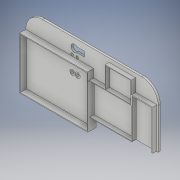
# Autodesk Inventor part: Base Plate 2
Saved by Autodesk Inventor 2018 (Build 220112000, 112)
## iProperties
Created: 2018-06-13
Part Number: Base Plate 2
Material: Generic
Document SubType Name: Modeling
Designer: brend
Density: 1 g/cm^3
Appearance: Default
Author: brend
Autodesk Inventor part; units mm, degrees
sketch "Sketch1" plane through (0, 0, 0) normal (0, 0, 1) x (1, 0, 0)
  line L0 (0, 87.3125) -> (163.83, 87.3125)
  line L1 (163.83, 87.3125) -> (163.83, 0)
  line L2 (163.83, 0) -> (0, 0)
  line L3 (0, 0) -> (0, 87.3125)
  dimension "d0" = 163.83
  dimension "d1" = 87.3125
  constraints: 8 end point, 2 parallel, 1 horizontal, 1 perpendicular
  measures "d0" distance between parallel lines of L1 L3
  measures "d1" distance between parallel lines of L2 L0
extrude "Extrusion1" add sketch "Sketch1" along normal blind 2.54
sketch "Sketch2" plane through (0, 0, 2.54) normal (0, 0, 1) x (1, 0, 0)
  point P0 (0, 0)
fillet "Fillet1" radius 20.6375 1 edges at (163.83, 87.3125, 1.27)
fillet "Fillet2" radius 20.6375 1 edges at (0, 87.3125, 1.27)
sketch "Sketch8" plane through (0, 0, 2.54) normal (0, 0, 1) x (1, 0, 0)
  point P0 (0, 0)
sketch "Sketch11" plane through (0, 0, 2.54) normal (0, 0, 1) x (1, 0, 0)
  point P0 (0, 0)
sketch "Sketch15" plane through (0, 0, 2.54) normal (0, 0, 1) x (1, 0, 0)
  line L0 (83.566, 56.2102) -> (136.1122, 56.2102)
  line L1 (136.1122, 56.2102) -> (136.1122, 16.51)
  line L2 (136.1122, 16.51) -> (83.566, 16.51)
  line L3 (83.566, 16.51) -> (83.566, 56.2102)
  line L4 (0, 0) -> (163.83, 0) projected
  line L5 (163.83, 0) -> (163.83, 66.675) projected
  dimension "d136" = 52.5463
  dimension "d137" = 16.51
  dimension "d151" = 39.7002
  dimension "d184" = 27.7177
  constraints: 8 end point, 2 parallel, 1 horizontal, 1 perpendicular
  measures "d136" distance between parallel lines of L1 L3
  measures "d137" distance between parallel lines of L4 L2
  measures "d151" distance between parallel lines of L2 L0
  measures "d184" distance between parallel lines of L5 L1
extrude "Extrusion6" add sketch "Sketch15" along normal blind 5.08
shell "Shell5" thickness 0.762 removed faces 1 at (101.0814, 42.9768, 7.62)
sketch "Sketch16" plane through (0, 0, 2.54) normal (0, 0, 1) x (1, 0, 0)
  line L0 (103.124, 82.5754) -> (135.89, 82.5754)
  line L1 (135.89, 82.5754) -> (135.89, 56.2102)
  line L2 (135.89, 56.2102) -> (103.124, 56.2102)
  line L3 (103.124, 56.2102) -> (103.124, 82.5754)
  arc A0 (163.83, 66.675) -> (143.1925, 87.3125) centre (143.1925, 66.675) ccw projected
  line L4 (136.1122, 56.2102) -> (83.566, 56.2102) projected
  point P0 (0, 0)
  dimension "d62" = 32.766
  dimension "d63" = 26.3652
  dimension "d183" = 27.94
  dimension "d231" = 0
  constraints: 8 end point, 2 parallel, 1 horizontal, 1 perpendicular
  measures "d62" distance of L1.end L2.end
  measures "d63" distance of L0.end L1.end
  measures "d231" distance between parallel lines of L4 L2
extrude "Extrusion7" add sketch "Sketch16" along normal blind 5.08
shell "Shell6" thickness 0.762 removed faces 1 at (124.968, 73.787, 7.62)
sketch "Sketch20" plane through (0, 0, 2.54) normal (0, 0, 1) x (1, 0, 0)
  circle A0 centre (60.325, 76.2) radius 4.445
  line L0 (0, 66.675) -> (0, 0) projected
  line L1 (103.124, 87.3125) -> (20.6375, 87.3125) projected
  point P0 (103.124, 82.5754)
  point P1 (20.6375, 87.3125)
  dimension "d77" = 8.89
  dimension "d138" = 60.325
  dimension "d150" = 11.1125
  constraints: 1 centre point
  measures "d77" diameter of A0
  measures "d138" distance from line of L0 A0.centre
  measures "d150" distance from line of L1 A0.centre
sketch "Sketch24" plane through (0, 0, 2.54) normal (0, 0, 1) x (1, 0, 0)
  line L0 (0, 0) -> (83.7565, 0)
  line L1 (83.7565, 0) -> (83.7565, 66.3575)
  line L2 (83.7565, 66.3575) -> (0, 66.3575)
  line L3 (0, 66.3575) -> (0, 0)
  line L4 (103.124, 87.3125) -> (20.6375, 87.3125) projected
  point P0 (103.124, 82.5754)
  point P1 (20.6375, 87.3125)
  dimension "d114" = 83.7565
  dimension "d210" = 20.955
  constraints: 8 end point, 2 parallel, 1 horizontal, 1 perpendicular
  measures "d114" distance of L2.end L1.end
  measures "d210" distance between parallel lines of L2 L4
extrude "Extrusion13" add sketch "Sketch24" along normal blind 7.62
sketch "Sketch25" plane through (0, 0, 2.54) normal (0, 0, 1) x (1, 0, 0)
  circle A0 centre (57.2977, 68.2625) radius 1.5875
  line L0 (0, 66.675) -> (0, 66.3575) projected
  circle A1 centre (63.6477, 68.2625) radius 1.5875
  line L1 (103.124, 87.3125) -> (20.6375, 87.3125) projected
  point P0 (0, 0)
  point P1 (103.124, 82.5754)
  point P2 (20.6375, 87.3125)
  dimension "d126" = 3.175
  dimension "d139" = 57.2977
  dimension "d141" = 6.35
  dimension "d149" = 19.05
  constraints: 2 centre point
  measures "d126" diameter of A0
  measures "d139" distance from line of L0 A0.centre
  measures "d141" distance of A1.centre A0.centre
  measures "d149" distance from line of L1 A0.centre
sketch "Sketch27" plane through (0, 0, 2.54) normal (0, 0, 1) x (1, 0, 0)
  line L0 (62.5475, 79.375) -> (72.7075, 79.375)
  line L1 (72.7075, 79.375) -> (72.7075, 73.025)
  line L2 (72.7075, 73.025) -> (62.5475, 73.025)
  line L3 (62.5475, 73.025) -> (62.5475, 79.375)
  arc A0 (20.6375, 87.3125) -> (0, 66.675) centre (20.6375, 66.675) ccw projected
  point P0 (0, 0)
  dimension "d181" = 41.91
  dimension "d182" = 10.16
  constraints: 8 end point, 2 parallel, 1 horizontal, 1 perpendicular
  measures "d181" distance from line of A0.centre L3
  measures "d182" distance between parallel lines of L1 L3
ref_plane "Work Plane1" through (0.508, 0.508, 2.286) normal (0, 0, 1) x (1, 0, 0)
sketch "Sketch28" plane through (0.508, 0.508, 2.286) normal (0, 0, 1) x (1, 0, 0)
  circle A0 centre (57.15, 48.7045) radius 1.5875
  circle A1 centre (56.7897, 67.7545) radius 1.5875 projected
  circle A2 centre (63.5, 48.7045) radius 1.5875
  circle A3 centre (62.992, 67.7545) radius 1.5875 projected
  point P0 (-0.508, -0.508)
  dimension "d154" = 19.05
  dimension "d155" = 3.175
  dimension "d156" = 19.05
  dimension "d157" = 6.35
  constraints: 2 centre point
  measures "d154" vertical distance of A0.centre A1.centre
  measures "d155" diameter of A2
  measures "d156" vertical distance of A2.centre A3.centre
  measures "d157" distance of A2.centre A0.centre
ref_plane "Work Plane2" through (0.508, 0.508, 2.286) normal (0, 0, 1) x (1, 0, 0)
sketch "Sketch29" plane through (0.508, 0.508, 2.286) normal (0, 0, 1) x (1, 0, 0)
  line L0 (82.7405, 64.7065) -> (0, 64.7065) projected
  line L1 (82.7405, 0) -> (0, 0) projected
  line L2 (0, 64.7065) -> (82.7405, 64.7065)
  line L3 (82.7405, 64.7065) -> (82.7405, 0)
  line L4 (82.7405, 0) -> (0, 0)
  line L5 (0, 0) -> (0, 64.7065)
  point P0 (-0.508, -0.508)
  point P1 (84.836, 62.484)
  constraints: 8 end point, 2 parallel, 1 horizontal, 1 perpendicular, 1 other
extrude "Extrusion16" add sketch "Sketch29" along normal blind 2.54
ref_plane "Work Plane3" through (0.508, 0.508, 4.826) normal (0, 0, 1) x (1, 0, 0)
sketch "Sketch30" plane through (0.508, 0.508, 4.826) normal (0, 0, 1) x (1, 0, 0)
  circle A0 centre (57.15, 48.7045) radius 3.175
  circle A1 centre (63.5, 48.7045) radius 3.175
  circle A2 centre (56.7897, 67.7545) radius 1.5875 projected
  circle A3 centre (62.992, 67.7545) radius 1.5875 projected
  point P0 (-0.508, -0.508)
  dimension "d162" = 6.35
  dimension "d163" = 19.05
  dimension "d164" = 19.05
  constraints: 2 centre point
  measures "d162" diameter of A1
  measures "d163" vertical distance of A2.centre A0.centre
  measures "d164" vertical distance of A3.centre A1.centre
sketch "Sketch33" plane through (20.6375, 86.5505, 0.762) normal (0, 0, 1) x (1, 0, 0)
  line L0 (63.6905, -69.2785) -> (63.6905, -31.1023) projected
  line L1 (114.7127, -69.2785) -> (63.6905, -69.2785) projected
  line L2 (63.6905, -31.1023) -> (114.7127, -31.1023)
  line L3 (114.7127, -31.1023) -> (114.7127, -69.2785)
  line L4 (114.7127, -69.2785) -> (63.6905, -69.2785)
  line L5 (63.6905, -69.2785) -> (63.6905, -31.1023)
  point P0 (-20.6375, -86.5505)
  constraints: 8 end point, 2 parallel, 1 horizontal, 1 perpendicular
extrude "Extrusion20" add sketch "Sketch33" along normal blind 1.778
sketch "Sketch34" plane through (0, 0, 0) normal (0, 0, -1) x (-1, 0, 0)
  line L0 (-163.83, 0) -> (0, 0)
  line L1 (0, 0) -> (0, 87.3125)
  line L2 (0, 87.3125) -> (-163.83, 87.3125)
  line L3 (-163.83, 87.3125) -> (-163.83, 0)
  point P0 (0, 0)
  constraints: 8 end point, 2 parallel, 1 horizontal, 1 perpendicular
extrude "Extrusion21" add sketch "Sketch34" against normal blind 2.54
extrude "Extrusion22" cut sketch "Sketch20" against normal blind 7.62
extrude "Extrusion23" cut sketch "Sketch25" against normal blind 7.62
extrude "Extrusion24" cut sketch "Sketch28" along normal mid plane 7.62 contours A0 | A2
extrude "Extrusion25" cut sketch "Sketch27" against normal blind 7.62
fillet "Fillet4" radius 20.6375 1 edges at (163.83, 87.3125, 1.27)
fillet "Fillet5" radius 20.6375 1 edges at (0, 87.3125, 1.27)
sketch "Sketch35" plane through (0, 0, 2.54) normal (0, 0, 1) x (1, 0, 0)
  line L0 (135.3502, 17.272) -> (84.328, 17.272) projected
  line L1 (135.3502, 17.272) -> (162.2742, 17.272)
  line L2 (162.2742, 17.272) -> (162.2742, 66.802)
  line L3 (162.2742, 66.802) -> (135.3502, 66.802)
  line L4 (135.3502, 66.802) -> (135.3502, 17.272)
  point P0 (0, 0)
  point P1 (85.344, 22.352)
  dimension "d199" = 26.924
  dimension "d200" = 49.53
  constraints: 8 end point, 2 parallel, 1 horizontal, 1 perpendicular, 1 other
  measures "d199" distance of L3.end L2.end
  measures "d200" distance of L2.end L1.end
extrude "Extrusion26" add sketch "Sketch35" along normal blind 5.08
sketch "Sketch36" plane through (0, 0, 7.62) normal (0, 0, 1) x (1, 0, 0)
  line L0 (136.6202, 65.532) -> (160.4327, 65.532)
  line L1 (160.4327, 65.532) -> (160.4327, 14.732)
  line L2 (160.4327, 14.732) -> (136.6202, 14.732)
  line L3 (136.6202, 14.732) -> (136.6202, 65.532)
  line L4 (135.3502, 55.4482) -> (135.3502, 17.272) projected
  line L5 (162.2742, 66.802) -> (135.89, 66.802) projected
  line L6 (136.1122, 17.272) -> (162.2742, 17.272) projected
  point P0 (0, 0)
  point P1 (135.3502, 66.802)
  dimension "d203" = 23.8125
  dimension "d204" = 1.27
  dimension "d205" = 1.27
  dimension "d207" = 50.8
  constraints: 8 end point, 2 parallel, 1 horizontal, 1 perpendicular
  measures "d203" distance of L1.end L2.end
  measures "d204" distance between parallel lines of L4 L3
  measures "d205" distance between parallel lines of L5 L0
  measures "d207" distance between parallel lines of L2 L0
extrude "Extrusion27" cut sketch "Sketch36" against normal blind 5.08
sketch "Sketch37" plane through (0, 0, 10.16) normal (0, 0, 1) x (1, 0, 0)
  line L0 (0.762, 3.048) -> (83.5152, 3.048)
  line L1 (83.5152, 3.048) -> (83.5152, 65.3859)
  line L2 (83.5152, 65.3859) -> (0.762, 65.386)
  line L3 (0.762, 65.386) -> (0.762, 3.048)
  line L4 (0, 66.3575) -> (0, 0) projected
  line L5 (0, 0) -> (83.7565, 0) projected
  dimension "d211" = 82.7532
  dimension "d212" = 62.3379
  dimension "d213" = 0.762
  dimension "d214" = 3.048
  constraints: 8 end point, 2 parallel, 1 horizontal, 1 perpendicular
  measures "d211" distance of L2.end L1.end
  measures "d212" distance of L1.end L0.end
  measures "d213" distance between parallel lines of L4 L3
  measures "d214" distance between parallel lines of L5 L0
extrude "Extrusion28" cut sketch "Sketch37" against normal blind 7.62
extrude "Extrusion29" cut sketch "Sketch30" against normal blind 2.54 contours A0 | A1
sketch "Sketch38" plane through (0, 0, 2.54) normal (0, 0, 1) x (1, 0, 0)
  line L0 (163.83, 0) -> (0, 0) projected
  line L1 (163.83, 0) -> (84.1375, 0)
  line L2 (84.1375, 0) -> (84.1375, 16.51)
  line L3 (84.1375, 16.51) -> (163.83, 16.51)
  line L4 (163.83, 16.51) -> (163.83, 0)
  dimension "d229" = 16.51
  constraints: 8 end point, 2 parallel, 1 horizontal, 1 perpendicular
  measures "d229" distance between parallel lines of L0 L3
extrude "Extrusion30" cut sketch "Sketch38" against normal blind 12.7
sketch "Sketch39" plane through (0, 0, 7.62) normal (0, 0, 1) x (1, 0, 0)
  line L0 (83.7565, 66.3575) -> (83.7565, 56.2102) projected
  line L1 (83.7565, 56.2102) -> (84.328, 56.2102)
  line L2 (84.328, 56.2102) -> (84.328, 0)
  line L3 (84.328, 0) -> (83.7565, 0)
  line L4 (83.7565, 0) -> (83.7565, 56.2102)
  line L5 (84.328, 17.272) -> (84.328, 55.4482) projected
  line L6 (83.7565, 0) -> (84.1375, 0) projected
  point P0 (0, 0)
  dimension "d221" = 0
  dimension "d230" = 0
  constraints: 8 end point, 2 parallel, 1 horizontal, 1 perpendicular
  measures "d221" distance between parallel lines of L5 L2
  measures "d230" distance between parallel lines of L6 L3
extrude "Extrusion31" add sketch "Sketch39" along normal blind 2.54 and the other way blind 7.62
sketch "Sketch40" plane through (0, 0, 10.16) normal (0, 0, 1) x (1, 0, 0)
  line L0 (84.328, 0) -> (84.328, 56.2102) projected
  line L1 (0, 0) -> (84.328, 0)
  line L2 (84.328, 0) -> (84.328, 2.032)
  line L3 (84.328, 2.032) -> (0, 2.032)
  line L4 (0, 2.032) -> (0, 0)
  line L5 (83.5152, 3.048) -> (0.762, 3.048) projected
  dimension "d226" = 1.016
  constraints: 8 end point, 2 parallel, 1 horizontal, 1 perpendicular, 1 point on line
  measures "d226" distance between parallel lines of L5 L3
extrude "Extrusion32" cut sketch "Sketch40" against normal blind 12.7
body "Solid1"
